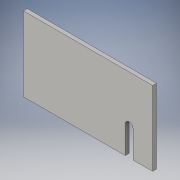
# Autodesk Inventor part: InsideRWall
Saved by Autodesk Inventor 2016 (Build 200138000, 138)
## iProperties
Created: 2016-05-30
Part Number: InsideRWall
Material: Generic
Document SubType Name: Modeling
Designer: cutrones
Density: 1 g/cm^3
Appearance: Default
Author: cutrones
Autodesk Inventor part; units mm, degrees
ref_plane "YZ Plane" through (0, 0, 0) normal (1, 0, 0) x (0, 1, 0)
ref_plane "XZ Plane" through (0, 0, 0) normal (0, 1, 0) x (-1, 0, 0)
ref_plane "XY Plane" through (0, 0, 0) normal (0, 0, 1) x (1, 0, 0)
sketch "Sketch1" plane through (0, 0, 0) normal (0, 0, 1) x (1, 0, 0)
  line L0 (0, 0) -> (419.1, 0)
  line L1 (419.1, 0) -> (419.1, 241.3)
  line L2 (419.1, 241.3) -> (0, 241.3)
  line L3 (0, 241.3) -> (0, 0)
  line L4 (419.1, 88.9) -> (342.9, 88.9)
  circle A0 centre (342.9, 88.9) radius 12.7
  line L5 (330.2, 88.9) -> (330.2, 0)
  line L6 (355.6, 88.9) -> (355.6, 0)
  dimension "d0" = 419.1
  dimension "d1" = 241.3
  dimension "d2" = 76.2
  dimension "d3" = 88.9
  dimension "d4" = 25.4
  dimension "d5" = 88.9
  constraints: 14 end point, 4 point on line, 3 perpendicular, 2 parallel, 2 point on circle, 1 centre point, 1 coincident, 1 horizontal, 1 tangent, 1 vertical
  measures "d0" distance of L2.end L1.end
  measures "d1" distance of L1.end L0.end
  measures "d2" distance of L4.start L4.end
  measures "d3" distance between parallel lines of L0 L4
  measures "d4" diameter of A0
  measures "d5" distance between parallel lines of L1 L5
extrude "Extrusion1" add sketch "Sketch1" along normal mid plane 12.7 contours L3 L2 L1 L4 A0 L5 L0 | L6 L4 L1 L0
equation "\"d0\" = Length"
equation "\"d1\" = Height"
equation "\"d6\" = Thickness"
equation "\"Length\" = 419.1"
equation "\"Height\" = 241.3"
equation "\"Thickness\" = 12.7"
body "Solid1"
